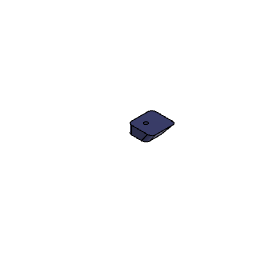
Standfuss_v56 (Autodesk Fusion 360 design; units mm, degrees)
Autodesk Fusion 360 part; units mm, degrees
sketch "Skizze1" plane through (0, 0, 0) normal (0, 0, -1) x (1, 0, 0)
  line L0 (-68.2, 73.2) -> (-68.2, -73.2)
  line L1 (-68.2, -73.2) -> (68.2, -73.2)
  line L2 (68.2, -73.2) -> (68.2, 73.2)
  line L3 (68.2, 73.2) -> (-68.2, 73.2)
  line L4 (-68.2, 73.2) -> (-48.2, 73.2)
  line L5 (-48.2, 73.2) -> (-48.2, 53.2)
  line L6 (-48.2, 53.2) -> (-68.2, 53.2)
  line L7 (-68.2, 53.2) -> (-68.2, 73.2)
  dimension "d802" = 20
  dimension "d803" = 20
  constraint horizontal L4
  constraint vertical L5
  constraint horizontal L6
  constraint vertical L7
  constraint coincident L0.start L3.end
  measures "d802" distance of L0.start L4.end
  measures "d803" distance of L0.start L6.end
ref_plane "Arbeitsebene1" through (0, 0, -7) normal (0, 0, -1) x (1, 0, 0)
sketch "Skizze2" plane through (0, 0, -7) normal (0, 0, -1) x (1, 0, 0)
  line L0 (-68.2, 73.2) -> (-48.2, 73.2)
  line L1 (-68.2, 53.2) -> (-68.2, 73.2)
  line L2 (-68.2, 73.2) -> (-53.2, 73.2)
  line L3 (-53.2, 73.2) -> (-53.2, 58.2)
  line L4 (-53.2, 58.2) -> (-68.2, 58.2)
  line L5 (-68.2, 58.2) -> (-68.2, 73.2)
  point P0 (-68.2, 73.2)
  dimension "d805" = 15
  dimension "d806" = 15
  constraint horizontal L2
  constraint vertical L3
  constraint horizontal L4
  constraint vertical L5
  constraint coincident P0 L0.start
  measures "d805" distance of P0 L2.end
  measures "d806" distance of P0 L4.end
loft "Erhebung1" add profiles "Skizze1", "Skizze2" section 1 contours L0 L3 L4 L5 L6 L7 section 2
sketch "Skizze3" plane through (0, 0, -7) normal (0, 0, -1) x (1, 0, 0)
  line L0 (-68.2, 58.2) -> (-53.2, 58.2)
  line L1 (-53.2, 58.2) -> (-53.2, 73.2)
  line L2 (-53.2, 73.2) -> (-68.2, 73.2)
  line L3 (-68.2, 73.2) -> (-68.2, 58.2)
  line L4 (-68.2, 73.2) -> (-53.2, 58.2) construction
  point P0 (-60.7, 65.7)
  constraint coincident L2.end L3.start
  constraint coincident L0.end L1.start
  constraint midpoint L4 P0
hole "Bohrung1" at (-60.7, -65.7, -7) direction (0, 0, 1) diameter 3 depth 7 tip angle 180 countersink diameter 6 countersink angle 90
fillet "Abrundung1" radius 3 4 edges at (-68.2, -73.2, -3.5) (-68.2, -55.7, -3.5) (-50.7, -55.7, -3.5) (-50.7, -73.2, -3.5)
